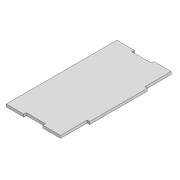
# Autodesk Inventor part: стенка 4
Saved by Autodesk Inventor 2021 (Build 250183000, 183)
## iProperties
Created: 2023-02-14
Part Number: стенка 4
Material: Типовые
Document SubType Name: Modeling
Designer: Tasya
Density: 1 g/cm^3
Appearance: По умолчанию
Author: Tasya
Autodesk Inventor part; units mm, degrees
ref_plane "YZ Plane" through (0, 0, 0) normal (1, 0, 0) x (0, 1, 0)
ref_plane "XZ Plane" through (0, 0, 0) normal (0, 1, 0) x (-1, 0, 0)
ref_plane "XY Plane" through (0, 0, 0) normal (0, 0, 1) x (1, 0, 0)
sketch "Эскиз1" plane through (0, 0, 0) normal (0, 1, 0) x (-1, 0, 0)
  line L0 (-42.5, 86.5) -> (42.5, 86.5)
  line L1 (42.5, 86.5) -> (42.5, -86.5)
  line L2 (42.5, -86.5) -> (-42.5, -86.5)
  line L3 (-42.5, -86.5) -> (-42.5, 86.5)
  line L4 (-42.5, 86.5) -> (42.5, -86.5) construction
  line L5 (42.5, 86.5) -> (-42.5, -86.5) construction
  line L6 (0, 0) -> (-44.5, 0) construction
  line L7 (-42.5, 45) -> (-46.5, 45)
  line L8 (-46.5, 45) -> (-46.5, -45)
  line L9 (-46.5, -45) -> (-42.5, -45)
  line L10 (-42.5, -45) -> (-42.5, 45)
  line L11 (-42.5, 45) -> (-46.5, -45) construction
  line L12 (-46.5, 45) -> (-42.5, -45) construction
  line L13 (-15, 82.5) -> (15, 82.5)
  line L14 (15, 82.5) -> (15, 86.5)
  line L15 (15, 86.5) -> (-15, 86.5)
  line L16 (-15, 86.5) -> (-15, 82.5)
  line L17 (-15, 82.5) -> (15, 86.5) construction
  line L18 (15, 82.5) -> (-15, 86.5) construction
  line L19 (0, -206.2504) -> (0, 0) construction
  line L20 (-15, -82.5) -> (15, -82.5)
  line L21 (15, -82.5) -> (15, -86.5)
  line L22 (-15, -86.5) -> (-15, -82.5)
  line L23 (15, -86.5) -> (-15, -86.5)
  point P0 (0, 0)
  point P1 (0, 0)
  point P2 (-10, -165.5)
  point P3 (-10, -255.5)
  point P4 (-44.5, 0)
  point P5 (-10, -45)
  point P6 (-10, 45)
  point P7 (0, 84.5)
  point P8 (-5, -342)
  point P9 (5, -342)
  point P10 (5, 342)
  point P11 (-5, 342)
  point P12 (0, 0)
  point P13 (5, 131)
  point P14 (-5, 131)
  point P15 (-10, 45)
  point P16 (-10, -45)
  point P17 (-5, -131)
  point P18 (5, -131)
  point P19 (0, 0)
  point P20 (-42.5, 45)
  dimension "d0" = 173
  dimension "d1" = 85
  dimension "d2" = 90
  dimension "d3" = 4
  dimension "d4" = 4
  dimension "d5" = 30
  constraints: 48 end point, 9 midpoint, 6 parallel, 4 horizontal, 4 symmetric about line, 3 perpendicular, 2 coincident, 2 collinear, 1 vertical, 1 other
  measures "d0" distance of L2.end L0.start
  measures "d1" distance between parallel lines of L3 L1
  measures "d2" distance of L7.end L8.end
  measures "d3" distance of L8.end L9.end
  measures "d4" distance of L15.end L13.start
  measures "d5" distance of L13.start L13.end
extrude "Выдавливание1" add sketch "Эскиз1" along normal blind 4 contours L0 L16 L13 L14 L1 L2 L21 L20 L22 L3 | L3 L9 L8 L7
